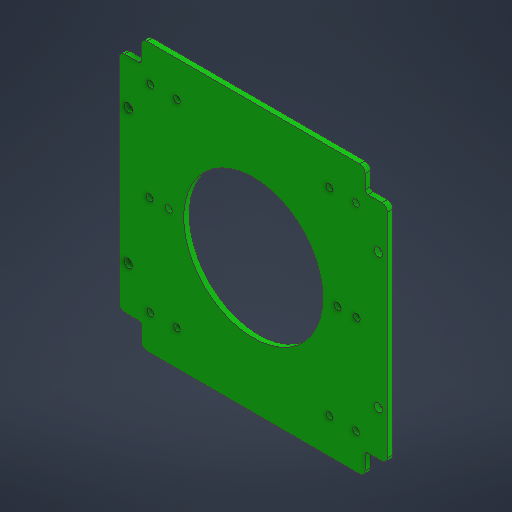
# Autodesk Inventor part: PCB
Saved by Autodesk Inventor 2026.1 (Build 301233020, 233B)
## iProperties
Created: 2025-11-06
Part Number: PCB
Material: Generic
Document SubType Name: Modeling
Designer: SPEL
Density: 1 g/cm^3
Appearance: Default
Author: SPEL
Autodesk Inventor part; units mm, degrees
ref_plane "YZ Plane" through (0, 0, 0) normal (1, 0, 0) x (0, 1, 0)
ref_plane "XZ Plane" through (0, 0, 0) normal (0, 1, 0) x (-1, 0, 0)
ref_plane "XY Plane" through (0, 0, 0) normal (0, 0, 1) x (1, 0, 0)
sketch "Sketch1" plane through (0, 0, 0) normal (0, 0, 1) x (1, 0, 0)
  circle A0 centre (0, 0) radius 25.5
  line L0 (-42, 41) -> (-47.2, 41)
  line L1 (-49.2, 39) -> (-49.2, -39)
  line L2 (42, -41) -> (47.2, -41)
  line L3 (49.2, -39) -> (49.2, 39)
  line L4 (49.2, 41) -> (-49.2, -41) construction
  line L5 (-49.2, 41) -> (49.2, -41) construction
  circle A1 centre (-45.8, 24.7) radius 1.6
  circle A2 centre (-45.8, -24.7) radius 1.6
  circle A3 centre (45.8, -24.7) radius 1.6
  circle A4 centre (45.8, 24.7) radius 1.6
  line L6 (39, -49.2) -> (-39, -49.2)
  line L7 (-41, 42) -> (-41, 47.2)
  line L8 (-39, 49.2) -> (39, 49.2)
  line L9 (41, -42) -> (41, -47.2)
  line L10 (41, -49.2) -> (-41, 49.2) construction
  line L11 (-41, -49.2) -> (41, 49.2) construction
  circle A5 centre (30.95, 0) radius 1.25
  circle A6 centre (37.95, 0) radius 1.25
  arc A7 (49.2, 39) -> (47.2, 41) centre (47.2, 39) ccw
  arc A8 (41, 47.2) -> (39, 49.2) centre (39, 47.2) ccw
  arc A9 (-39, 49.2) -> (-41, 47.2) centre (-39, 47.2) ccw
  arc A10 (-47.2, 41) -> (-49.2, 39) centre (-47.2, 39) ccw
  arc A11 (-49.2, -39) -> (-47.2, -41) centre (-47.2, -39) ccw
  arc A12 (-41, -47.2) -> (-39, -49.2) centre (-39, -47.2) ccw
  arc A13 (39, -49.2) -> (41, -47.2) centre (39, -47.2) ccw
  arc A14 (47.2, -41) -> (49.2, -39) centre (47.2, -39) ccw
  arc A15 (-42, 41) -> (-41, 42) centre (-42, 42) ccw
  arc A16 (42, -41) -> (41, -42) centre (42, -42) ccw
  line L12 (47.2, 41) -> (42, 41)
  line L13 (41, 47.2) -> (41, 42)
  line L14 (-41, -47.2) -> (-41, -42)
  line L15 (-47.2, -41) -> (-42, -41)
  arc A17 (-41, -42) -> (-42, -41) centre (-42, -42) ccw
  arc A18 (41, 42) -> (42, 41) centre (42, 42) ccw
  circle A19 centre (37.7, 36.2) radius 1.25
  circle A20 centre (27.95, 36.2) radius 1.25
  line L16 (0, 0) -> (74.274, 0)
  line L17 (0, 0) -> (0, 66.673)
  circle A21 centre (37.7, -36.2) radius 1.25
  circle A22 centre (27.95, -36.2) radius 1.25
  circle A23 centre (-37.7, 36.2) radius 1.25
  circle A24 centre (-27.95, 36.2) radius 1.25
  circle A25 centre (-37.7, -36.2) radius 1.25
  circle A26 centre (-27.95, -36.2) radius 1.25
  circle A27 centre (-30.95, 0) radius 1.25
  circle A28 centre (-37.95, 0) radius 1.25
  point P0 (41, -41)
  point P1 (-41, -41)
  point P2 (-41, 41)
  point P3 (41, 41)
  dimension "d0" = 51
  dimension "d1" = 98.4
  dimension "d2" = 82
  dimension "d29" = 82
  dimension "d50" = 3.2
  dimension "d52" = 3.2
  dimension "d53" = 3.2
  dimension "d55" = 3.2
  dimension "d57" = 49.4
  dimension "d58" = 49.4
  dimension "d59" = 91.6
  dimension "d60" = 91.6
  dimension "d61" = 45.8
  dimension "d62" = 45.8
  dimension "d63" = 24.7
  dimension "d64" = 24.7
  dimension "d67" = 82
  dimension "d68" = 98.4
  dimension "d73" = 2.5
  dimension "d74" = 2.5
  dimension "d77" = 11.25
  dimension "d78" = 18.25
  dimension "d79" = 2
  dimension "d80" = 1
  dimension "d81" = 1
  dimension "d82" = 1
  dimension "d83" = 2.5
  dimension "d84" = 2.5
  dimension "d85" = 13
  dimension "d86" = 13
  dimension "d87" = 11.5
  dimension "d88" = 21.25
  constraints: 36 end point, 29 centre point, 24 point on circle, 24 tangent, 20 point on line, 8 equal radius, 8 symmetric about line, 4 horizontal, 4 midpoint, 4 parallel, 4 perpendicular, 2 vertical, 1 coincident, 8 other
  measures "d0" diameter of A0
  measures "d1" distance of L5.end L4.end
  measures "d2" distance of L4.end L5.start
  measures "d29" distance of L5.end L4.start
  measures "d50" diameter of A1
  measures "d52" diameter of A2
  measures "d53" diameter of A3
  measures "d55" diameter of A4
  measures "d57" distance of A2.centre A1.centre
  measures "d58" distance of A3.centre A4.centre
  measures "d59" distance of A4.centre A1.centre
  measures "d60" distance of A3.centre A2.centre
  measures "d61" horizontal distance of A1.centre point (0, 0)
  measures "d62" horizontal distance of point (0, 0) A2.centre
  measures "d63" vertical distance of point (0, 0) A1.centre
  measures "d64" vertical distance of point (0, 0) A4.centre
  measures "d67" distance of L10.end L11.end
  measures "d68" distance of L11.start L10.end
  measures "d73" diameter of A5
  measures "d74" diameter of A6
  measures "d77" distance from line of A6.centre L3
  measures "d78" distance from line of L3 A5.centre
  measures "d79" radius of A7
  measures "d80" radius of A15
  measures "d81" radius of A16
  measures "d82" radius of A17
  measures "d83" diameter of A20
  measures "d84" diameter of A19
  measures "d85" distance from line of L8 A19.centre
  measures "d86" distance from line of L8 A20.centre
  measures "d87" distance from line of L3 A19.centre
  measures "d88" distance from line of L3 A20.centre
extrude "Extrusión15" add sketch "Sketch1" along normal blind 2 contours L16 A5 A6 L3 A14 L2 A16 L9 A13 L6 A12 L14 A17 L15 A11 L1 A10 L0 A15 L7 A9 L8 L17 A0 | A0 L17 L8 A8 L13 A18 L12 A7 L3 L16 A6 A5
equation "\"d52\" = d50"
equation "\"d53\" = d54"
equation "\"d55\" = d56"
equation "\"d58\" = d57"
equation "\"d60\" = d59"
equation "\"d61\" = 0.5 * d59"
equation "\"d62\" = d61"
equation "\"d63\" = 0.5 * d57"
equation "\"d64\" = d63"
equation "\"d74\" = d73"
equation "\"d83\" = d73"
equation "\"d84\" = d73"
equation "\"d86\" = d85"
equation "\"d54\" = 3.2"
equation "\"d56\" = 3.2"
